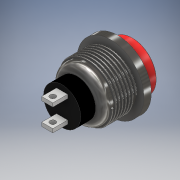
# Autodesk Inventor part: PushButton
Saved by Autodesk Inventor 2018 (Build 220112000, 112)
## iProperties
Created: 2017-12-07
Part Number: PushButton
Material: Generic
Document SubType Name: Modeling
Designer: Julian
Density: 1 g/cm^3
Appearance: Default
Author: Julian
Autodesk Inventor part; units mm, degrees
ref_plane "YZ Plane" through (0, 0, 0) normal (1, 0, 0) x (0, 1, 0)
ref_plane "XZ Plane" through (0, 0, 0) normal (0, 1, 0) x (-1, 0, 0)
ref_plane "XY Plane" through (0, 0, 0) normal (0, 0, 1) x (1, 0, 0)
sketch "Sketch1" plane through (0, 0, 0) normal (0, 1, 0) x (-1, 0, 0)
  circle A0 centre (0, 0) radius 9
  dimension "d0" = 18
  constraints: 1 centre point, 1 coincident
  measures "d0" diameter of A0
extrude "Extrusion1" add sketch "Sketch1" along normal blind 2
sketch "Sketch2" plane through (0, 2, 0) normal (0, 1, 0) x (1, 0, 0)
  circle A0 centre (0, 0) radius 6.5
  dimension "d3" = 13
  constraints: 1 centre point, 1 coincident
  measures "d3" diameter of A0
extrude "Extrusion2" add sketch "Sketch2" along normal blind 4
sketch "Sketch3" plane through (0, 0, 0) normal (0, -1, 0) x (1, 0, 0)
  circle A0 centre (0, 0) radius 7
  dimension "d6" = 14
  constraints: 1 centre point, 1 coincident
  measures "d6" diameter of A0
extrude "Extrusion3" add sketch "Sketch3" along normal blind 7
sketch "Sketch5" plane through (0, 0, 0) normal (0, 0, 1) x (1, 0, 0)
  line L0 (-7, -7) -> (7, -7) projected
  line L1 (0, -7) -> (7, -7)
  line L2 (7, -7) -> (7, -6.5)
  line L3 (7, -6.5) -> (7.5, -6.5)
  line L4 (7.5, -6.5) -> (7.5, -7)
  line L5 (7.5, -7) -> (7, -7)
  line L6 (0, -7) -> (0, -7.9183)
  point P0 (0, 0)
  constraints: 12 end point, 3 perpendicular, 2 vertical, 1 horizontal
coil "Coil1" sketch "Sketch5" operation add axis through (0, -7, 0) along (0, 1, 0) pitch 0.9 turns 7 hand right
fillet "Fillet1" radius 0.25 28 edges at (0, -6.775, -7.5) (0, -6.325, 7.5) (0, -5.875, -7.5) (0, -5.425, 7.5) (0, -4.975, -7.5) (0, -4.525, 7.5) (0, -4.075, -7.5) (0, -3.625, 7.5) (0, -3.175, -7.5) (0, -2.725, 7.5) (0, -2.275, -7.5) (0, -1.825, 7.5) (0, -1.375, -7.5) (0, -0.925, 7.5) (0, -6.275, -7.5) (0, -5.825, 7.5) (0, -5.375, -7.5) (0, -4.925, 7.5) (0, -4.475, -7.5) (0, -4.025, 7.5) (0, -3.575, -7.5) (0, -3.125, 7.5) (0, -2.675, -7.5) (0, -2.225, 7.5) (0, -1.775, -7.5) (0, -1.325, 7.5) (0, -0.875, -7.5) (0, -0.425, 7.5)
sketch "Sketch6" plane through (0, -7, 0) normal (0, -1, 0) x (1, 0, 0)
  line L0 (7.25, 0) -> (7, 0) projected
  circle A0 centre (0, 0) radius 7
  constraints: 1 coincident, 1 horizontal alignment, 2 other
extrude "Extrusion4" add sketch "Sketch6" along normal blind 2
fillet "Fillet2" radius 2 1 edges at (-7, -9, 0)
sketch "Sketch7" plane through (0, -9, 0) normal (0, -1, 0) x (1, 0, 0)
  circle A0 centre (0, 0) radius 5
  constraints: 1 centre point, 1 coincident
extrude "Extrusion5" add sketch "Sketch7" along normal blind 4
fillet "Fillet3" radius 0.2 1 edges at (-6.5, 6, 0)
sketch "Sketch8" plane through (0, -13, 0) normal (0, -1, 0) x (1, 0, 0)
  line L0 (0, -2.5) -> (-1.5, -2.5)
  line L1 (-1.5, -2.5) -> (1.5, -2.5)
  line L2 (1.5, -2.5) -> (1.5, -3.5)
  line L3 (1.5, -3.5) -> (-1.5, -3.5)
  line L4 (-1.5, -3.5) -> (-1.5, -2.5)
  line L5 (0, 2.5) -> (1.5, 2.5)
  line L6 (1.5, 2.5) -> (1.5, 3.5)
  line L7 (1.5, 3.5) -> (0, 3.5)
  line L8 (0, 2.5) -> (-1.5, 2.5)
  line L9 (-1.5, 2.5) -> (-1.5, 3.5)
  line L10 (-1.5, 3.5) -> (0, 3.5)
  line L11 (1.5, 3.5) -> (-1.5, 3.5)
  line L12 (-1.5, 3.5) -> (-1.5, 2.5)
  line L13 (-1.5, 2.5) -> (1.5, 2.5)
  line L14 (1.5, 2.5) -> (1.5, 3.5)
  point P0 (0, 0)
  constraints: 30 end point, 6 parallel, 5 horizontal, 4 perpendicular
extrude "Extrusion6" add sketch "Sketch8" along normal blind 4
sketch "Sketch9" plane through (-1.5, -13, 3.5) normal (0, 0, 1) x (1, 0, 0)
  circle A0 centre (1.5, -2.5) radius 0.75
  point P0 (1.5, 13)
  point P1 (3, -4)
  constraints: 1 centre point
extrude "Extrusion7" cut sketch "Sketch9" against normal blind 10
body "Solid1"
